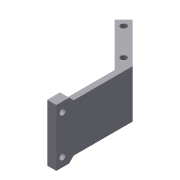
# Autodesk Inventor part: Knee - Front
Saved by Autodesk Inventor 2011 (Build 150239000, 239)
## iProperties
Created: 2010-11-21
Part Number: Knee - Front
Document SubType Name: Modeling
Designer: Milton
Density: 2.71 g/cm^3
Mass: 12.6425 g
Surface Area: 35.3697 cm^2
Volume: 4.66513 cm^3
Material: Aluminum-6061
Author: Milton
Autodesk Inventor part; units mm, degrees
ref_plane "YZ Plane" through (0, 0, 0) normal (1, 0, 0) x (0, 1, 0)
sketch "Sketch1" plane through (0, 0, 0) normal (0, 0, 1) x (1, 0, 0)
  circle A0 centre (27.3252, 37.9057) radius 1.35
  line L0 (28.532, 3.2058) -> (28.532, 8.8058)
  line L1 (28.532, 8.8058) -> (30.032, 8.8058)
  line L2 (10.8964, 50.3787) -> (14.8568, 54.3379)
  line L3 (14.8568, 54.3379) -> (32.532, 36.6578)
  line L4 (32.532, 36.6578) -> (32.532, 3.2058)
  line L5 (28.532, 3.2058) -> (32.532, 3.2058)
  line L6 (30.032, 31.2378) -> (10.8964, 50.3787)
  line L7 (30.032, 8.8058) -> (30.032, 31.2378)
  circle A1 centre (15.306, 49.9282) radius 1.35
  point P0 (0, 0)
  dimension "d1" = 5.6
  dimension "d26" = 1.5
  dimension "d36" = 4
  dimension "d38" = 2.7
  constraints: 16 end point, 4 perpendicular, 2 centre point, 1 horizontal, 1 vertical
  measures "d1" distance of L0.start L0.end
  measures "d26" distance of L0.end L1.end
  measures "d36" distance of L0.start L4.end
  measures "d38" diameter of A1
ref_plane "Work Plane1" through (25.095, 32.5645, 21) normal (0, 0, -1) x (-0.707008, 0.7072056, 0)
extrude "Extrusion3" add sketch "Sketch1" along normal up to surface (21 mm away)
sketch "Sketch3" plane through (32.532, 3.2058, 0) normal (1, 0, 0) x (0, 0, -1)
  circle A0 centre (-19, 2.8) radius 1.35
  circle A1 centre (-2, 2.8) radius 1.35
  circle A2 centre (-2, 2.8) radius 1.35 projected
  circle A3 centre (-19, 2.8) radius 1.35 projected
  point P0 (0, -3.2058)
  dimension "d41" = 2.7
  dimension "d42" = 2.7
  constraints: 2 centre point, 2 concentric
  measures "d41" diameter of A1
  measures "d42" diameter of A0
extrude "Extrusion4" cut sketch "Sketch3" against normal through all
sketch "Sketch4" plane through (32.532, 3.2058, 0) normal (1, 0, 0) x (0, 0, -1)
  circle A0 centre (-19, 2.8) radius 1.35 projected
  circle A1 centre (-2, 2.8) radius 1.35 projected
  line L0 (-21, 0) -> (-21, 33.452) projected
  line L1 (0, 0) -> (0, 33.452) projected
  line L2 (-23, 5.6) -> (2, 5.6)
  line L3 (2, 5.6) -> (2, 0)
  line L4 (2, 0) -> (-23, 0)
  line L5 (-23, 0) -> (-23, 5.6)
  point P0 (0, -3.2058)
  dimension "d48" = 2
  dimension "d49" = 2
  constraints: 8 end point, 2 parallel, 1 horizontal, 1 perpendicular
  measures "d48" distance between parallel lines of L3 L1
  measures "d49" distance between parallel lines of L0 L5
ref_plane "Work Plane2" through (28.532, -58.9903, -31.7364) normal (1, 0, 0) x (0, 1, 0)
extrude "Extrusion5" add sketch "Sketch4" against normal up to surface (4 mm away)
chamfer "Chamfer1" distance 2 angle 45 2 edges at (31.282, 8.8058, 21) (31.282, 8.8058, 0)
body "Solid2"
